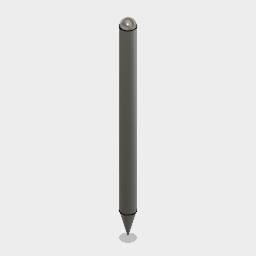
cld2 (Autodesk Fusion 360 design; units mm, degrees)
Autodesk Fusion 360 part; units mm, degrees
cylinder "圆柱体基本要素1" add diameter 8 height 100 placed x (1, 0, 0) y (0, 0, -1) z (0, 1, 0) at (0, 0, 0) makes body 1
sphere "球体基本要素1" add diameter 8 placed x (0, 0, -1) y (0, 1, 0) z (1, 0, 0) at (0, 84, 42) separate body makes body 2
move_body "对齐1" bodies 2 to x (1, 0, 0) y (0, 0, 1) z (0, -1, 0) at (0, 142, -84)
sketch "草图3" plane through (0, 0, 0) normal (1, 0, 0) x (0, 0, -1)
  line L0 (-25, 0) -> (-40, 0)
  line L1 (-40, 0) -> (-40, 4)
  line L2 (-25, 0) -> (-40, 4)
  dimension "d4" = 4
  measures "d4" distance of L0.end L1.end
revolve "旋转1" add sketch "草图3" angle 360 about axis through (0, 0, 25) along (0, 0, 1) separate body makes body 3
move_face "MoveFace1" to x (1, 0, 0) y (0, 1, 0) z (0, 0, 1) at (16.6586, -111.9007, 0) 1 faces at (3.3689, -1.3222, 38.5714) on bodies 3
move_body "对齐2" bodies 3 to x (-1, 0, 0) y (0, 0, 1) z (0, 1, 0) at (16.6586, -40, 111.9007)
combine "合并1" operation add target body 2 tool bodies 1 3
sketch "草图4" plane through (0, 0, 0) normal (1, 0, 0) x (0, 0, -1)
